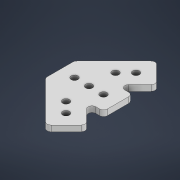
# Autodesk Inventor part: 45 degree angle bracket
Saved by Autodesk Inventor 2022 (Build 260153000, 153)
## iProperties
Created: 2022-01-17
Part Number: 45 degree angle bracket
Material: Generic
Document SubType Name: Modeling
Designer: izack
Density: 1 g/cm^3
Appearance: Default
Author: izack
Autodesk Inventor part; units mm, degrees
ref_plane "YZ Plane" through (0, 0, 0) normal (1, 0, 0) x (0, 1, 0)
ref_plane "XZ Plane" through (0, 0, 0) normal (0, 1, 0) x (-1, 0, 0)
ref_plane "XY Plane" through (0, 0, 0) normal (0, 0, 1) x (1, 0, 0)
sketch "Sketch1" plane through (0, 0, 0) normal (0, 1, 0) x (-1, 0, 0)
  line L0 (0, 0) -> (0, 15)
  line L1 (0, 15) -> (-30, 15)
  line L2 (-30, 15) -> (-30, 0)
  line L3 (-30, 0) -> (0, 0)
  line L4 (0, 0) -> (-21.2132, -21.2132)
  line L5 (0, 0) -> (30, 0) construction
  line L6 (-21.2132, -21.2132) -> (-31.8198, -10.6066)
  line L7 (-31.8198, -10.6066) -> (-21.2132, 0)
  line L8 (0, 15) -> (-21.2132, 36.2132)
  line L9 (0, 15) -> (30, 15) construction
  line L10 (-21.2132, 36.2132) -> (-31.8198, 25.6066)
  line L11 (-31.8198, 25.6066) -> (-21.2132, 15)
  dimension "d0" = 15
  dimension "d1" = 30
  dimension "d2" = 30
  dimension "d3" = 135
  dimension "d4" = 15
  dimension "d5" = 30
  dimension "d6" = 135
  constraints: 24 end point, 7 perpendicular, 2 equal length, 2 horizontal, 2 point on line, 2 vertical
  measures "d0" distance of L0.start L0.end
  measures "d1" distance of L0.end L1.end
  measures "d2" distance of L0.start L4.end
  measures "d3" angle of L4 L5
  measures "d4" distance of L4.end L6.end
  measures "d5" distance of L0.end L8.end
  measures "d6" angle of L9 L8
extrude "Extrusion1" add sketch "Sketch1" along normal blind 3
sketch "Sketch2" plane through (0, 3, 0) normal (0, 1, 0) x (1, 0, 0)
  circle A0 centre (21.2132, -25.6066) radius 1.75
  circle A1 centre (15.9099, -20.3033) radius 1.75
  circle A2 centre (15, -7.5) radius 1.75
  circle A3 centre (21.2132, 10.6066) radius 1.75
  circle A4 centre (15.9099, 5.3033) radius 1.75
  circle A5 centre (7.5, -7.5) radius 1.75
  circle A6 centre (22.5, -7.5) radius 1.75
  line L0 (31.8198, -25.6066) -> (21.2132, -15) projected
  line L1 (30, 0) -> (21.2132, 0) projected
  line L2 (21.2132, 0) -> (31.8198, 10.6066) projected
  line L3 (21.2132, -36.2132) -> (31.8198, -25.6066) projected
  line L4 (30, -15) -> (30, 0) projected
  line L5 (0, 0) -> (0, -15) projected
  line L6 (31.8198, 10.6066) -> (21.2132, 21.2132) projected
  dimension "d9" = 3.5
  dimension "d10" = 3.5
  dimension "d11" = 3.5
  dimension "d12" = 3.5
  dimension "d13" = 3.5
  dimension "d14" = 3.5
  dimension "d15" = 3.5
  dimension "d16" = 7.5
  dimension "d18" = 7.5
  dimension "d19" = 7.5
  dimension "d20" = 7.5
  dimension "d21" = 7.5
  dimension "d22" = 7.5
  dimension "d23" = 7.5
  dimension "d24" = 7.5
  dimension "d26" = 15
  dimension "d27" = 7.5
  dimension "d28" = 15
  dimension "d29" = 7.5
  dimension "d30" = 15
  dimension "d31" = 7.5
  constraints: 7 centre point
  measures "d9" diameter of A0
  measures "d10" diameter of A1
  measures "d11" diameter of A2
  measures "d12" diameter of A3
  measures "d13" diameter of A4
  measures "d14" diameter of A5
  measures "d15" diameter of A6
  measures "d16" distance from line of L0 A0.centre
  measures "d18" distance from line of L0 A1.centre
  measures "d19" distance from line of L1 A5.centre
  measures "d20" distance from line of L1 A2.centre
  measures "d21" distance from line of L1 A6.centre
  measures "d22" distance from line of L2 A4.centre
  measures "d23" distance from line of L2 A3.centre
  measures "d24" distance from line of L3 A0.centre
  measures "d26" distance from line of L3 A1.centre
  measures "d27" distance from line of L4 A6.centre
  measures "d28" distance from line of L4 A2.centre
  measures "d29" distance from line of L5 A5.centre
  measures "d30" distance from line of L6 A4.centre
  measures "d31" distance from line of L6 A3.centre
extrude "Extrusion2" cut sketch "Sketch2" against normal through all
fillet "Fillet1" radius 2 10 edges at (21.2132, 1.5, -21.2132) (31.8198, 1.5, -10.6066) (21.2132, 1.5, 0) (30, 1.5, 0) (30, 1.5, 15) (21.2132, 1.5, 15) (31.8198, 1.5, 25.6066) (21.2132, 1.5, 36.2132) (0, 1.5, 15) (0, 1.5, 0)
equation "\"d16\" = a"
equation "\"d18\" = a"
equation "\"d19\" = a"
equation "\"d20\" = a"
equation "\"d21\" = a"
equation "\"d22\" = a"
equation "\"d23\" = a"
equation "\"d24\" = a"
equation "\"d27\" = a"
equation "\"d29\" = a"
equation "\"d31\" = a"
equation "\"a\" = 7.5"
body "Solid1"
